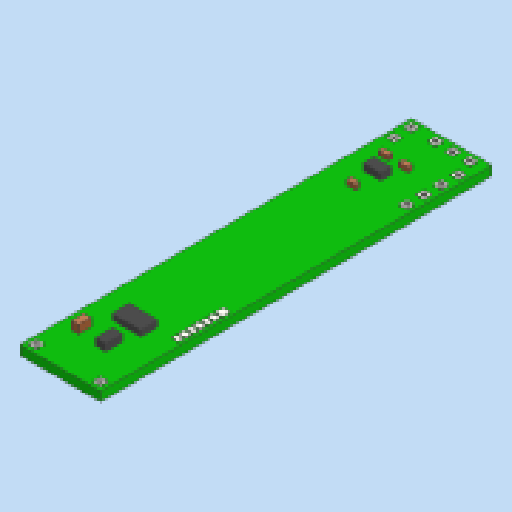
# Autodesk Inventor part: MCU_PCB
Saved by Autodesk Inventor 2024 (Build 280153000, 153)
## iProperties
Created: 2025-02-15
Part Number: MCU_PCB
Material: Generic
Document SubType Name: Modeling
Designer: XxPan
Density: 1 g/cm^3
Appearance: Default
Author: XxPan
Autodesk Inventor part; units mm, degrees
ref_plane "YZ Plane" through (0, 0, 0) normal (1, 0, 0) x (0, 1, 0)
ref_plane "XZ Plane" through (0, 0, 0) normal (0, 1, 0) x (-1, 0, 0)
ref_plane "XY Plane" through (0, 0, 0) normal (0, 0, 1) x (1, 0, 0)
sketch "Sketch1" plane through (0, 0, 0) normal (0, 1, 0) x (-1, 0, 0)
  line L0 (7, 34) -> (-7, 34)
  line L1 (-7, 34) -> (-7, -34)
  line L2 (-7, -34) -> (7, -34)
  line L3 (7, -34) -> (7, 34)
  line L4 (9.8, 0) -> (-9.8, 0) construction
  line L5 (0, -47.6) -> (0, 47.6) construction
  point P0 (0, 0)
  point P1 (7, 0)
  point P2 (0, 34)
  dimension "d0" = 14
  dimension "d1" = 68
  constraints: 8 end point, 2 midpoint, 2 parallel, 2 point on line, 1 horizontal, 1 perpendicular
  measures "d0" distance of L2.end L1.end
  measures "d1" distance of L2.end L0.start
extrude "fr4" add sketch "Sketch1" along normal mid plane 1.6
sketch "Sketch5" plane through (-7, 0.8, -34) normal (0, 1, 0) x (1, 0, 0)
  line L0 (12.3, -0.7) -> (10.9, -0.7)
  line L1 (10.9, -0.7) -> (10.9, -2.1)
  line L2 (10.9, -2.1) -> (12.3, -2.1)
  line L3 (12.3, -2.1) -> (12.3, -0.7)
  line L4 (13.3, -3.7) -> (11.9, -3.7)
  line L5 (11.9, -3.7) -> (11.9, -5.1)
  line L6 (11.9, -5.1) -> (13.3, -5.1)
  line L7 (13.3, -5.1) -> (13.3, -3.7)
  line L8 (13.3, -6.7) -> (11.9, -6.7)
  line L9 (11.9, -6.7) -> (11.9, -8.1)
  line L10 (11.9, -8.1) -> (13.3, -8.1)
  line L11 (13.3, -8.1) -> (13.3, -6.7)
  line L12 (13.3, -9.7) -> (11.9, -9.7)
  line L13 (11.9, -9.7) -> (11.9, -11.1)
  line L14 (11.9, -11.1) -> (13.3, -11.1)
  line L15 (13.3, -11.1) -> (13.3, -9.7)
  line L16 (13.3, -12.7) -> (11.9, -12.7)
  line L17 (11.9, -12.7) -> (11.9, -14.1)
  line L18 (11.9, -14.1) -> (13.3, -14.1)
  line L19 (13.3, -14.1) -> (13.3, -12.7)
  line L20 (9.3, -0.7) -> (7.9, -0.7)
  line L21 (7.9, -0.7) -> (7.9, -2.1)
  line L22 (7.9, -2.1) -> (9.3, -2.1)
  line L23 (9.3, -2.1) -> (9.3, -0.7)
  line L24 (6.3, -0.7) -> (4.9, -0.7)
  line L25 (4.9, -0.7) -> (4.9, -2.1)
  line L26 (4.9, -2.1) -> (6.3, -2.1)
  line L27 (6.3, -2.1) -> (6.3, -0.7)
  line L28 (2.1, -0.7) -> (0.7, -0.7)
  line L29 (0.7, -0.7) -> (0.7, -2.1)
  line L30 (0.7, -2.1) -> (2.1, -2.1)
  line L31 (2.1, -2.1) -> (2.1, -0.7)
  line L32 (2.1, -3.7) -> (0.7, -3.7)
  line L33 (0.7, -3.7) -> (0.7, -5.1)
  line L34 (0.7, -5.1) -> (2.1, -5.1)
  line L35 (2.1, -5.1) -> (2.1, -3.7)
  line L36 (14, -68) -> (14, 0) projected
  line L37 (14, 0) -> (0, 0) projected
  line L38 (0, 0) -> (0, -68) projected
  line L39 (13.3, -65.9) -> (11.9, -65.9)
  line L40 (11.9, -65.9) -> (11.9, -67.3)
  line L41 (11.9, -67.3) -> (13.3, -67.3)
  line L42 (13.3, -67.3) -> (13.3, -65.9)
  line L43 (2.1, -65.9) -> (0.7, -65.9)
  line L44 (0.7, -65.9) -> (0.7, -67.3)
  line L45 (0.7, -67.3) -> (2.1, -67.3)
  line L46 (2.1, -67.3) -> (2.1, -65.9)
  line L47 (0, -68) -> (14, -68) projected
  point P0 (7, -34)
  dimension "d23" = 1.4
  dimension "d24" = 1.4
  dimension "d25" = 1.4
  dimension "d26" = 1.4
  dimension "d27" = 1.4
  dimension "d28" = 1.4
  dimension "d29" = 1.4
  dimension "d30" = 1.4
  dimension "d31" = 1.4
  dimension "d32" = 1.4
  dimension "d33" = 1.4
  dimension "d34" = 1.4
  dimension "d35" = 1.4
  dimension "d36" = 1.4
  dimension "d37" = 1.4
  dimension "d38" = 1.4
  dimension "d39" = 1.4
  dimension "d40" = 1.4
  dimension "d41" = 0.7
  dimension "d42" = 1.7
  dimension "d43" = 0.7
  dimension "d44" = 0.7
  dimension "d45" = 3.7
  dimension "d47" = 3
  dimension "d48" = 3
  dimension "d49" = 3
  dimension "d50" = 3
  dimension "d51" = 3
  dimension "d52" = 1.4
  dimension "d53" = 1.4
  dimension "d54" = 1.4
  dimension "d55" = 1.4
  dimension "d56" = 0.7
  dimension "d57" = 0.7
  dimension "d58" = 0.7
  constraints: 88 end point, 22 parallel, 11 horizontal, 11 perpendicular, 9 collinear
  measures "d23" distance of L2.end L1.end
  measures "d24" distance of L1.end L0.end
  measures "d25" distance of L6.end L5.end
  measures "d26" distance of L5.end L4.end
  measures "d27" distance of L10.end L9.end
  measures "d28" distance of L9.end L8.end
  measures "d29" distance of L14.end L13.end
  measures "d30" distance of L13.end L12.end
  measures "d31" distance of L18.end L17.end
  measures "d32" distance of L17.end L16.end
  measures "d33" distance of L22.end L21.end
  measures "d34" distance of L21.end L20.end
  measures "d35" distance of L26.end L25.end
  measures "d36" distance of L25.end L24.end
  measures "d37" distance of L30.end L29.end
  measures "d38" distance of L29.end L28.end
  measures "d39" distance of L34.end L33.end
  measures "d40" distance of L33.end L32.end
  measures "d41" distance between parallel lines of L36 L7
  measures "d42" distance between parallel lines of L36 L3
  measures "d43" distance between parallel lines of L37 L0
  measures "d44" distance between parallel lines of L38 L29
  measures "d45" distance between parallel lines of L37 L32
  measures "d47" distance between parallel lines of L23 L3
  measures "d48" distance between parallel lines of L27 L23
  measures "d49" distance between parallel lines of L8 L4
  measures "d50" distance between parallel lines of L12 L8
  measures "d51" distance between parallel lines of L16 L12
  measures "d52" distance of L41.end L40.end
  measures "d53" distance of L45.end L44.end
  measures "d54" distance of L44.end L43.end
  measures "d55" distance of L39.end L40.end
  measures "d56" distance between parallel lines of L36 L42
  measures "d57" distance between parallel lines of L47 L41
  measures "d58" distance between parallel lines of L38 L44
extrude "connector pads" add sketch "Sketch5" along normal blind 0.1 and the other way blind 1.7 contours L3 L2 L1 L0 | L7 L6 L5 L4 | L11 L10 L9 L8 | L15 L14 L13 L12 | L19 L18 L17 L16 | L23 L22 L21 L20 | L27 L26 L25 L24 | L31 L30 L29 L28 | L35 L34 L33 L32 | L42 L41 L40 L39 | L46 L45 L44 L43
sketch "Sketch6" plane through (-7, 0.9, -34) normal (0, 1, 0) x (1, 0, 0)
  line L0 (13.3, -5.1) -> (13.3, -3.7) projected
  line L1 (13.3, -3.7) -> (11.9, -3.7) projected
  line L2 (12.3, -2.1) -> (12.3, -0.7) projected
  line L3 (0.7, -0.7) -> (0.7, -2.1) projected
  line L4 (11.9, -67.3) -> (13.3, -67.3) projected
  point P0 (7, -34)
  point P1 (12.6, -4.4)
  point P2 (12.6, -7.4)
  point P3 (12.6, -10.4)
  point P4 (12.6, -13.4)
  point P5 (11.6, -1.4)
  point P6 (8.6, -1.4)
  point P7 (5.6, -1.4)
  point P8 (1.4, -1.4)
  point P9 (1.4, -4.4)
  point P10 (1.4, -66.6)
  point P11 (12.6, -66.6)
  dimension "d70" = 0.7
  dimension "d71" = 3
  dimension "d72" = 3
  dimension "d73" = 3
  dimension "d74" = 3
  dimension "d75" = 3
  dimension "d76" = 3
  dimension "d77" = 0.7
  dimension "d78" = 0.7
  dimension "d79" = 0.7
  dimension "d80" = 0.7
  constraints: 6 vertical alignment, 5 horizontal alignment
  measures "d70" distance from line of L0 point (12.6, -4.4)
  measures "d71" distance of point (12.6, -7.4) point (12.6, -4.4)
  measures "d72" distance of point (12.6, -10.4) point (12.6, -7.4)
  measures "d73" distance of point (12.6, -13.4) point (12.6, -10.4)
  measures "d74" distance of point (8.6, -1.4) point (11.6, -1.4)
  measures "d75" distance of point (8.6, -1.4) point (5.6, -1.4)
  measures "d76" distance of point (1.4, -4.4) point (1.4, -1.4)
  measures "d77" distance from line of L1 point (12.6, -4.4)
  measures "d78" distance from line of L2 point (11.6, -1.4)
  measures "d79" distance from line of L3 point (1.4, -1.4)
  measures "d80" distance from line of L4 point (12.6, -66.6)
hole "connector holes" at (5.6, 0.9, -29.6) at (5.6, 0.9, -26.6) at (5.6, 0.9, -23.6) at (5.6, 0.9, -20.6) at (4.6, 0.9, -32.6) at (1.6, 0.9, -32.6) at (-1.4, 0.9, -32.6) at (-5.6, 0.9, -32.6) at (-5.6, 0.9, -29.6) at (-5.6, 0.9, 32.6) at (5.6, 0.9, 32.6) direction (0, -1, 0) diameter 0.8 end through all
sketch "Sketch7" plane through (0, 0.8, 0) normal (0, 1, 0) x (1, 0, 0)
  line L0 (5.15, -19.9) -> (6.45, -19.9)
  line L1 (6.45, -19.9) -> (6.45, -18.95)
  line L2 (6.45, -18.95) -> (5.15, -18.95)
  line L3 (5.15, -18.95) -> (5.15, -19.9)
  line L4 (5.15, -18.63) -> (6.45, -18.63)
  line L5 (6.45, -18.63) -> (6.45, -17.68)
  line L6 (6.45, -17.68) -> (5.15, -17.68)
  line L7 (5.15, -17.68) -> (5.15, -18.63)
  line L8 (5.15, -17.36) -> (6.45, -17.36)
  line L9 (6.45, -17.36) -> (6.45, -16.41)
  line L10 (6.45, -16.41) -> (5.15, -16.41)
  line L11 (5.15, -16.41) -> (5.15, -17.36)
  line L12 (5.15, -16.09) -> (6.45, -16.09)
  line L13 (6.45, -16.09) -> (6.45, -15.14)
  line L14 (6.45, -15.14) -> (5.15, -15.14)
  line L15 (5.15, -15.14) -> (5.15, -16.09)
  line L16 (5.15, -14.82) -> (6.45, -14.82)
  line L17 (6.45, -14.82) -> (6.45, -13.87)
  line L18 (6.45, -13.87) -> (5.15, -13.87)
  line L19 (5.15, -13.87) -> (5.15, -14.82)
  line L20 (5.15, -13.55) -> (6.45, -13.55)
  line L21 (6.45, -13.55) -> (6.45, -12.6)
  line L22 (6.45, -12.6) -> (5.15, -12.6)
  line L23 (5.15, -12.6) -> (5.15, -13.55)
  line L24 (5.15, -12.28) -> (6.45, -12.28)
  line L25 (6.45, -12.28) -> (6.45, -10.88)
  line L26 (6.45, -10.88) -> (5.15, -10.88)
  line L27 (5.15, -10.88) -> (5.15, -12.28)
  line L28 (7, -34) -> (7, 34) projected
  line L29 (-7, -34) -> (7, -34) projected
  point P0 (0, 0)
  dimension "d81" = 1.3
  dimension "d82" = 0.95
  dimension "d83" = 1.27
  dimension "d84" = 1.27
  dimension "d85" = 1.27
  dimension "d86" = 1.27
  dimension "d88" = 1.27
  dimension "d89" = 1.27
  dimension "d90" = 0.95
  dimension "d91" = 0.95
  dimension "d92" = 0.95
  dimension "d93" = 0.95
  dimension "d94" = 0.95
  dimension "d95" = 1.4
  dimension "d96" = 0.55
  dimension "d97" = 14.1
  constraints: 56 end point, 14 parallel, 12 collinear, 7 horizontal, 7 perpendicular
  measures "d81" distance of L0.start L0.end
  measures "d82" distance of L2.end L0.start
  measures "d83" distance between parallel lines of L4 L0
  measures "d84" distance between parallel lines of L8 L4
  measures "d85" distance between parallel lines of L12 L8
  measures "d86" distance between parallel lines of L16 L12
  measures "d88" distance between parallel lines of L20 L16
  measures "d89" distance between parallel lines of L24 L20
  measures "d90" distance of L6.end L4.start
  measures "d91" distance of L10.end L8.start
  measures "d92" distance of L14.end L12.start
  measures "d93" distance of L18.end L16.start
  measures "d94" distance of L22.end L20.start
  measures "d95" distance of L26.end L24.start
  measures "d96" distance between parallel lines of L1 L28
  measures "d97" distance between parallel lines of L0 L29
extrude "programming interface" add sketch "Sketch7" along normal blind 0.1
sketch "Sketch8" plane through (0, 0.8, 0) normal (0, 1, 0) x (1, 0, 0)
  line L0 (-2.7, -22.3) -> (2.3, -22.3)
  line L1 (2.3, -22.3) -> (2.3, -19.3)
  line L2 (2.3, -19.3) -> (-2.7, -19.3)
  line L3 (-2.7, -19.3) -> (-2.7, -22.3)
  line L4 (-7, 34) -> (-7, -34) projected
  line L5 (-7, -34) -> (7, -34) projected
  point P0 (0, 0)
  dimension "d100" = 5
  dimension "d101" = 3
  dimension "d102" = 4.3
  dimension "d103" = 11.7
  constraints: 8 end point, 2 parallel, 1 horizontal, 1 perpendicular
  measures "d100" distance of L2.end L1.end
  measures "d101" distance of L1.end L0.end
  measures "d102" distance between parallel lines of L4 L3
  measures "d103" distance between parallel lines of L5 L0
extrude "accelerometer" add sketch "Sketch8" along normal blind 1
sketch "Sketch9" plane through (0, 0.8, 0) normal (0, 1, 0) x (1, 0, 0)
  line L0 (-4.8, -27.3) -> (-3.5, -27.3)
  line L1 (-3.5, -27.3) -> (-3.5, -25.1)
  line L2 (-3.5, -25.1) -> (-4.8, -25.1)
  line L3 (-4.8, -25.1) -> (-4.8, -27.3)
  line L4 (-7, 34) -> (-7, -34) projected
  line L5 (-7, -34) -> (7, -34) projected
  point P0 (0, 0)
  dimension "d106" = 1.3
  dimension "d107" = 2.2
  dimension "d108" = 2.2
  dimension "d109" = 6.7
  constraints: 8 end point, 2 parallel, 1 horizontal, 1 perpendicular
  measures "d106" distance of L2.end L1.end
  measures "d107" distance of L1.end L0.end
  measures "d108" distance between parallel lines of L4 L3
  measures "d109" distance between parallel lines of L5 L0
extrude "0804 cap" add sketch "Sketch9" along normal blind 1.4
sketch "Sketch10" plane through (0, 0.8, 0) normal (0, 1, 0) x (1, 0, 0)
  line L0 (-0.3, -27.6) -> (1.5, -27.6)
  line L1 (1.5, -27.6) -> (1.5, -24.6)
  line L2 (1.5, -24.6) -> (-0.3, -24.6)
  line L3 (-0.3, -24.6) -> (-0.3, -27.6)
  line L4 (-7, -34) -> (7, -34) projected
  line L5 (7, -34) -> (7, 34) projected
  line L6 (-3.3, 22) -> (-0.3, 22)
  line L7 (-0.3, 22) -> (-0.3, 23.8)
  line L8 (-0.3, 23.8) -> (-3.3, 23.8)
  line L9 (-3.3, 23.8) -> (-3.3, 22)
  line L10 (-7, 34) -> (-7, -34) projected
  line L11 (7, 34) -> (-7, 34) projected
  point P0 (0, 0)
  dimension "d112" = 1.8
  dimension "d113" = 3
  dimension "d114" = 6.4
  dimension "d115" = 5.5
  dimension "d118" = 3
  dimension "d119" = 1.8
  dimension "d120" = 3.7
  dimension "d121" = 10.2
  constraints: 16 end point, 4 parallel, 2 horizontal, 2 perpendicular
  measures "d112" distance of L2.end L1.end
  measures "d113" distance of L1.end L0.end
  measures "d114" distance between parallel lines of L4 L0
  measures "d115" distance between parallel lines of L5 L1
  measures "d118" distance of L8.end L7.end
  measures "d119" distance of L7.end L6.end
  measures "d120" distance between parallel lines of L10 L9
  measures "d121" distance between parallel lines of L11 L8
extrude "regulators" add sketch "Sketch10" along normal blind 1.2 contours L3 L2 L1 L0 | L9 L8 L7 L6
sketch "Sketch11" plane through (0, 0.8, 0) normal (0, 1, 0) x (1, 0, 0)
  line L0 (-4.3, 25.6) -> (-2.7, 25.6)
  line L1 (-2.7, 25.6) -> (-2.7, 26.4)
  line L2 (-2.7, 26.4) -> (-4.3, 26.4)
  line L3 (-4.3, 26.4) -> (-4.3, 25.6)
  line L4 (-2.7, 18.4) -> (-1.1, 18.4)
  line L5 (-1.1, 18.4) -> (-1.1, 19.2)
  line L6 (-1.1, 19.2) -> (-2.7, 19.2)
  line L7 (-2.7, 19.2) -> (-2.7, 18.4)
  line L8 (-0.8, 25.6) -> (0.8, 25.6)
  line L9 (0.8, 25.6) -> (0.8, 26.4)
  line L10 (0.8, 26.4) -> (-0.8, 26.4)
  line L11 (-0.8, 26.4) -> (-0.8, 25.6)
  line L12 (-7, 34) -> (-7, -34) projected
  line L13 (7, 34) -> (-7, 34) projected
  point P0 (0, 0)
  point P1 (0, 26.4)
  point P2 (-3.5, 26.4)
  point P3 (-1.9, 18.4)
  point P4 (-2.7, 18.8)
  point P5 (-4.3, 26)
  dimension "d122" = 1.6
  dimension "d123" = 0.8
  dimension "d124" = 1.6
  dimension "d125" = 0.8
  dimension "d126" = 1.6
  dimension "d127" = 0.8
  dimension "d129" = 7
  dimension "d130" = 3.5
  dimension "d131" = 5.1
  dimension "d132" = 15.2
  dimension "d133" = 8
  constraints: 24 end point, 6 parallel, 5 midpoint, 3 horizontal, 3 perpendicular, 1 collinear
  measures "d122" distance of L2.end L1.end
  measures "d123" distance of L1.end L0.end
  measures "d124" distance of L6.end L5.end
  measures "d125" distance of L5.end L4.end
  measures "d126" distance of L10.end L9.end
  measures "d127" distance of L9.end L8.end
  measures "d129" distance from line of L12 point (0, 26.4)
  measures "d130" distance of point (-3.5, 26.4) point (0, 26.4)
  measures "d131" distance from line of L12 point (-1.9, 18.4)
  measures "d132" distance from line of L13 point (-2.7, 18.8)
  measures "d133" distance from line of L13 point (-4.3, 26)
extrude "0603 cap" add sketch "Sketch11" along normal blind 0.8
sketch "Sketch12" plane through (0, 0.8, 0) normal (0, 1, 0) x (1, 0, 0)
  line L0 (-1.3, -18.25) -> (-0.3, -18.25)
  line L1 (-0.3, -18.25) -> (-0.3, -17.75)
  line L2 (-0.3, -17.75) -> (-1.3, -17.75)
  line L3 (-1.3, -17.75) -> (-1.3, -18.25)
  line L4 (3.15, -21.7) -> (3.65, -21.7)
  line L5 (3.65, -21.7) -> (3.65, -20.7)
  line L6 (3.65, -20.7) -> (3.15, -20.7)
  line L7 (3.15, -20.7) -> (3.15, -21.7)
  line L8 (7, -34) -> (7, 34) projected
  line L9 (-7, -34) -> (7, -34) projected
  line L10 (-7, 34) -> (-7, -34) projected
  point P0 (0, 0)
  point P1 (3.4, -21.7)
  point P2 (3.65, -21.2)
  point P3 (-0.8, -17.75)
  point P4 (-1.3, -18)
  dimension "d136" = 1
  dimension "d137" = 0.5
  dimension "d138" = 0.5
  dimension "d139" = 1
  dimension "d140" = 3.6
  dimension "d141" = 12.8
  dimension "d142" = 6.2
  dimension "d143" = 16
  constraints: 16 end point, 4 midpoint, 4 parallel, 2 horizontal, 2 perpendicular
  measures "d136" distance of L2.end L1.end
  measures "d137" distance of L1.end L0.end
  measures "d138" distance of L6.end L5.end
  measures "d139" distance of L5.end L4.end
  measures "d140" distance from line of L8 point (3.4, -21.7)
  measures "d141" distance from line of L9 point (3.65, -21.2)
  measures "d142" distance from line of L10 point (-0.8, -17.75)
  measures "d143" distance from line of L9 point (-1.3, -18)
extrude "0402 res" add sketch "Sketch12" along normal blind 0.4
sketch "Sketch13" plane through (0, 0.8, 0) normal (0, 1, 0) x (1, 0, 0)
  line L0 (1.9, -24.25) -> (2.9, -24.25)
  line L1 (2.9, -24.25) -> (2.9, -23.75)
  line L2 (2.9, -23.75) -> (1.9, -23.75)
  line L3 (1.9, -23.75) -> (1.9, -24.25)
  line L4 (-7, -34) -> (7, -34) projected
  line L5 (7, -34) -> (7, 34) projected
  point P0 (0, 0)
  point P1 (2.9, -24)
  point P2 (2.4, -24.25)
  dimension "d146" = 1
  dimension "d147" = 0.5
  dimension "d148" = 10
  dimension "d149" = 4.6
  constraints: 8 end point, 2 midpoint, 2 parallel, 1 horizontal, 1 perpendicular
  measures "d146" distance of L2.end L1.end
  measures "d147" distance of L1.end L0.end
  measures "d148" distance from line of L4 point (2.9, -24)
  measures "d149" distance from line of L5 point (2.4, -24.25)
extrude "0402 cap" add sketch "Sketch13" along normal blind 0.4
equation "\"d84\" = d83"
equation "\"d85\" = d83"
equation "\"d86\" = d83"
equation "\"d88\" = d83"
equation "\"d89\" = d83"
equation "\"d90\" = d82"
equation "\"d91\" = d82"
equation "\"d92\" = d82"
equation "\"d93\" = d82"
equation "\"d94\" = d82"
body "Solid1"
